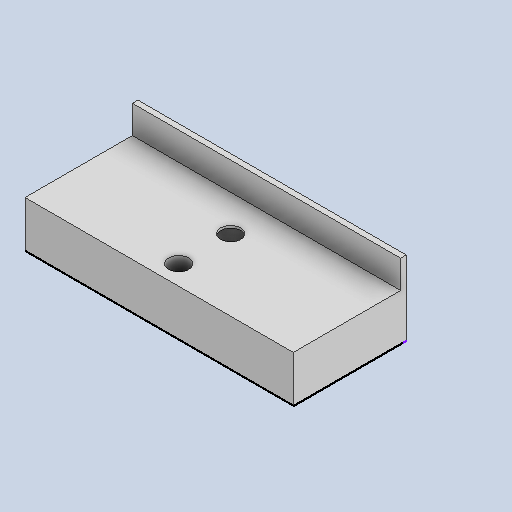
# Autodesk Inventor part: RotationMounttoPolarisPinAdapter
Saved by Autodesk Inventor 2024.2 (Build 282272000, 272)
## iProperties
Created: 2024-01-05
Part Number: RotationMounttoPolarisPinAdapter
Material: Generic
Document SubType Name: Modeling
Designer: monolithic
Density: 1 g/cm^3
Appearance: Default
Author: monolithic
Autodesk Inventor part; units mm, degrees
ref_plane "YZ Plane" through (0, 0, 0) normal (1, 0, 0) x (0, 1, 0)
ref_plane "XZ Plane" through (0, 0, 0) normal (0, 1, 0) x (-1, 0, 0)
ref_plane "XY Plane" through (0, 0, 0) normal (0, 0, 1) x (1, 0, 0)
sketch "Sketch1" plane through (0, 0, 0) normal (0, 1, 0) x (-1, 0, 0)
  line L0 (0, 0) -> (30.48, 0)
  line L1 (30.48, 0) -> (-30.48, 0)
  line L2 (-30.48, 0) -> (-30.48, -15.748)
  line L3 (-30.48, -15.748) -> (30.48, -15.748)
  line L4 (30.48, -15.748) -> (30.48, 0)
  line L5 (30.48, -15.748) -> (30.48, -15.494)
  line L6 (30.48, -15.494) -> (-30.48, -15.494)
  line L7 (0, 0) -> (0, -7.366)
  circle A0 centre (0, -7.366) radius 2.286
  line L8 (30.48, 0) -> (30.48, 8.89)
  line L9 (30.48, 8.89) -> (-30.48, 8.89)
  line L10 (-30.48, 8.89) -> (-30.48, 0)
  line L11 (30.48, 0) -> (-30.48, 0)
  line L12 (0, 0) -> (0, 4.445)
  circle A1 centre (0, 4.445) radius 2.286
  line L13 (30.48, -15.748) -> (-30.48, -15.748)
  line L14 (-30.48, -15.748) -> (-30.48, -16.7568)
  line L15 (-30.48, -16.7568) -> (30.48, -16.7568)
  line L16 (30.48, -16.7568) -> (30.48, -15.748)
  dimension "d0" = 30.48
  dimension "d1" = 60.96
  dimension "d2" = 15.748
  dimension "d3" = 0.254
  dimension "d4" = 7.366
  dimension "d5" = 4.572
  dimension "d14" = 8.89
  dimension "d15" = 4.572
  constraints: 34 end point, 8 perpendicular, 3 point on line, 3 vertical, 2 centre point, 2 coincident, 2 horizontal, 2 parallel
  measures "d0" distance of L0.start L0.end
  measures "d1" distance of L0.end L1.end
  measures "d2" distance of L1.end L2.end
  measures "d3" distance of L3.end L5.end
  measures "d4" distance of L0.start L7.end
  measures "d5" diameter of A0
  measures "d14" distance of L0.end L8.end
  measures "d15" diameter of A1
extrude "Extrusion1" add sketch "Sketch1" along normal blind 10.414 contours L0 L4 L6 L2 L1
extrude "Extrusion2" add sketch "Sketch1" along normal blind 16.764 contours L4 L3 L2 L6 | L16 L15 L14 L3
sketch "Sketch2" plane through (0, 0, 0) normal (0, -1, 0) x (1, 0, 0)
  line L0 (0, 0) -> (0, -7.366)
  circle A0 centre (0, -7.366) radius 3.81
  dimension "d10" = 7.366
  dimension "d11" = 7.62
  constraints: 2 end point, 1 centre point, 1 coincident, 1 vertical
  measures "d10" distance of L0.start L0.end
  measures "d11" diameter of A0
extrude "Extrusion3" cut sketch "Sketch2" against normal blind 9.906
extrude "Extrusion4" add sketch "Sketch1" along normal blind 10.414 contours L1 L10 L9 L8 L0
sketch "Sketch3" plane through (0, 0, 0) normal (0, -1, 0) x (1, 0, 0)
  line L0 (0, 4.5142) -> (5.0038, 4.5142)
  line L1 (0, 4.5142) -> (-5.0038, 4.5142)
  circle A0 centre (5.0038, 4.5142) radius 1.0109
  circle A1 centre (-5.0038, 4.5142) radius 1.0109
  point P0 (0, 0)
  dimension "d18" = 5.0038
  dimension "d19" = 5.0038
  dimension "d20" = 2.0218
  dimension "d21" = 2.0218
  constraints: 4 end point, 2 centre point, 2 coincident, 2 horizontal
  measures "d18" distance of L0.start L0.end
  measures "d19" distance of L0.start L1.end
  measures "d20" diameter of A0
  measures "d21" diameter of A1
extrude "Extrusion5" cut sketch "Sketch3" against normal blind 4.445
body "Solid1"
